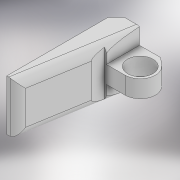
# Autodesk Inventor part: Foot
Saved by Autodesk Inventor 2022 (Build 260153000, 153)
## iProperties
Created: 2022-02-26
Part Number: Foot
Material: Generic
Document SubType Name: Modeling
Designer: joshw
Density: 1 g/cm^3
Appearance: Default
Author: joshw
Autodesk Inventor part; units mm, degrees
ref_plane "YZ Plane" through (0, 0, 0) normal (1, 0, 0) x (0, 1, 0)
ref_plane "XZ Plane" through (0, 0, 0) normal (0, 1, 0) x (-1, 0, 0)
ref_plane "XY Plane" through (0, 0, 0) normal (0, 0, 1) x (1, 0, 0)
sketch "Sketch1" plane through (0, 0, 0) normal (0, 1, 0) x (-1, 0, 0)
  circle A0 centre (49.0175, 1.0065) radius 3.6
  line L0 (58.9307, -3.2235) -> (48.4307, -3.2235)
  line L1 (58.9307, -3.2235) -> (58.9307, 22.7221)
  line L2 (58.9307, 22.7221) -> (56.4307, 22.7221)
  line L3 (56.4307, 22.7221) -> (53.9307, 7.6757)
  line L4 (53.9307, 7.6757) -> (53.9307, 4.6065)
  line L5 (53.9307, 4.6065) -> (49.0175, 4.6065)
  line L6 (53.4307, -3.2235) -> (53.4307, 4.6065)
  line L7 (46.6824, -1.7334) -> (48.4307, -3.2235)
  circle A1 centre (49.0175, 1.0065) radius 3
  point P0 (0, 0)
  dimension "d0" = 5.5
  dimension "d1" = 5
  dimension "d2" = 2.5
  dimension "d3" = 10.5
  dimension "d4" = 7.2
  dimension "d5" = 6
  dimension "d14" = 4.23
  constraints: 16 end point, 2 centre point, 2 point on circle, 2 point on line, 2 tangent, 1 coincident, 1 horizontal, 1 parallel, 1 perpendicular, 1 vertical
  measures "d0" distance between parallel lines of L6 L1
  measures "d1" distance between parallel lines of L4 L1
  measures "d2" distance of L1.end L2.end
  measures "d3" distance of L0.start L0.end
  measures "d4" diameter of A0
  measures "d5" diameter of A1
  measures "d14" distance from line of L0 A0.centre
extrude "Extrusion1" add sketch "Sketch1" along normal mid plane 4.1
extrude "Extrusion2" add sketch "Sketch1" along normal mid plane 12 contours L5 L4 L3 L2 L1 L0 L6
fillet "Fillet1" radius 2 3 edges at (-56.4307, 0, 22.7221) (-55.1807, 6, 15.1989) (-55.1807, -6, 15.1989)
chamfer "Chamfer1" distance 2 angle 45 1 edges at (-58.9307, 0, -3.2235)
body "Solid1"
